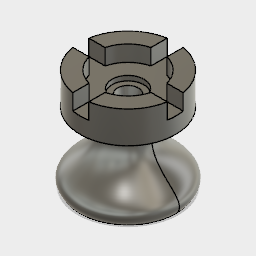
烛台 v0 (Autodesk Fusion 360 design; units mm, degrees)
Autodesk Fusion 360 part; units mm, degrees
sketch "草图1" plane through (0, 0, 0) normal (0, 0, 1) x (1, 0, 0)
  line L0 (0, 0) -> (30, 0)
  line L1 (0, 0) -> (0, 40)
  line L2 (0, 40) -> (15, 40)
  spline S0 degree 5 poles (15, 40) (14.8683, 39.1944) (14.6561, 37.6045) (14.4916, 35.283) (14.5823, 32.3156) (15.2193, 28.8245) (16.3774, 25.5572) (18.0321, 22.5165) (20.1227, 19.6996) (22.5351, 17.0933) (25.0868, 14.6699) (27.5575, 12.3937) (29.7153, 10.2259) (31.3448, 8.1296) (32.2727, 6.0736) (32.4056, 4.0384) (31.8532, 2.4191) (31.0692, 1.2082) (30.3836, 0.4025) (30, 0) knots 0 0 0 0 0 0 0.066667 0.133333 0.2 0.266667 0.333333 0.4 0.466667 0.533333 0.6 0.666667 0.733333 0.8 0.866667 0.933333 1 1 1 1 1 1
  line L3 (0, 40) -> (20, 40)
  line L4 (20, 40) -> (20, 43)
  line L5 (20, 43) -> (0, 43)
  line L6 (0, 43) -> (0, 40)
  circle A0 centre (20, 40) radius 2
  point P0 (20, 20)
  point P1 (31.5061, 7.5429)
  dimension "d1" = 15
  dimension "d2" = 40
  dimension "d3" = 30
  dimension "d4" = 3
  dimension "d5" = 20
  dimension "d6" = 4
  measures "d1" distance of L1.end L2.end
  measures "d2" distance of L0.start L1.end
  measures "d3" distance of L0.start L0.end
  measures "d4" distance of L1.end L5.end
  measures "d5" distance of L4.end L5.end
  measures "d6" diameter of A0
revolve "旋转1" add sketch "草图1" angle 360 about axis through (0, 0, 0) along (0, 1, 0) makes body 1
cylinder "圆柱体基本要素1" add diameter 60 height 20 placed x (1, 0, 0) y (0, 0, -1) z (0, 1, 0) at (0, 43, 0) bodies 1
shell "抽壳1" thickness 10 removed faces 1 at (6.9346, 63, 6.2102) on bodies 1
box "长方体基本要素2" add length 70 width 10 height 10 placed x (0, 0, 1) y (1, 0, 0) z (0, 1, 0) at (-110, 0, -50) separate body makes body 2
copy_body "复制和粘贴实体1" bodies 2 makes body 3
move_body "移动1" bodies 3 to x (0, 0, 1) y (0, 1, 0) z (-1, 0, 0) at (-160, 0, 60)
move_body "对齐1" bodies 3 to x (1, 0, 0) y (0, 1, 0) z (0, 0, 1) at (0, 0, 0)
move_body "对齐2" bodies 3 to x (-1, 0, 0) y (0, 1, 0) z (0, 0, -1) at (-250, 0, -60)
combine "合并1" operation add target body 2 tool bodies 3
move_body "对齐3" bodies 2 to x (1, 0, 0) y (0, 1, 0) z (0, 0, 1) at (105, 53, 15)
combine "合并2" operation cut target body 1 tool bodies 2
